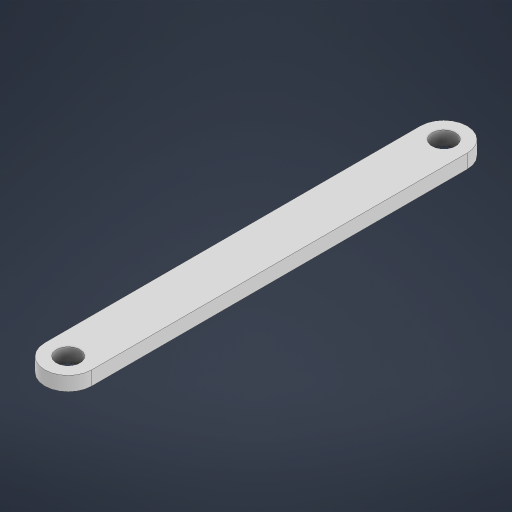
# Autodesk Inventor part: FP V2 Spring beam Short
Saved by Autodesk Inventor 2023.6 (Build 276521000, 521)
## iProperties
Created: 2026-02-24
Part Number: FP V2 Spring beam Short
Material: Generic
Document SubType Name: Modeling
Designer: user
Density: 1 g/cm^3
Appearance: Default
Author: user
Autodesk Inventor part; units mm, degrees
ref_plane "YZ Plane" through (0, 0, 0) normal (1, 0, 0) x (0, 1, 0)
ref_plane "XZ Plane" through (0, 0, 0) normal (0, 1, 0) x (-1, 0, 0)
ref_plane "XY Plane" through (0, 0, 0) normal (0, 0, 1) x (1, 0, 0)
sketch "Sketch1" plane through (0, 0, 0) normal (0, 1, 0) x (-1, 0, 0)
  line L0 (5, 40) -> (-5, 40)
  line L1 (-5, 40) -> (-5, -40)
  line L2 (-5, -40) -> (5, -40)
  line L3 (5, -40) -> (5, 40)
  line L4 (5, 40) -> (-5, -40) construction
  line L5 (-5, 40) -> (5, -40) construction
  circle A0 centre (0, 40) radius 5
  circle A1 centre (0, -40) radius 5
  circle A2 centre (0, 40) radius 2.5
  circle A3 centre (0, -40) radius 2.5
  point P0 (0, 0)
  point P1 (5, 40)
  point P2 (-5, 40)
  point P3 (5, -40)
  dimension "d0" = 80
  dimension "d1" = 10
  dimension "d2" = 5
  dimension "d3" = 5
  constraints: 12 end point, 4 midpoint, 3 centre point, 2 coincident, 2 parallel, 1 horizontal, 1 perpendicular, 1 tangent, 3 other
  measures "d0" distance between parallel lines of L2 L0
  measures "d1" distance between parallel lines of L1 L3
  measures "d2" diameter of A2
  measures "d3" diameter of A3
extrude "Extrusion1" add sketch "Sketch1" along normal blind 3 contours A0 L0 A2 | L0 A2 A0 | L3 A1 L1 A0 | A1 L2 A3 | L2 A3 A1
body "Solid1"
